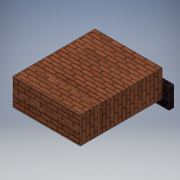
# Autodesk Inventor part: Камин
Saved by Autodesk Inventor 2019 (Build 230136000, 136)
## iProperties
Created: 2018-09-19
Part Number: Камин
Material: Кирпич, обычный, коричневый
Document SubType Name: Modeling
Designer: Андреев Н.Л.
Density: 1.95 g/cm^3
Appearance: Равномерная кладка — непрерывный ряд — оранжевый
Author: Андреев Н.Л.
Autodesk Inventor part; units mm, degrees
ref_plane "YZ Plane" through (0, 0, 0) normal (1, 0, 0) x (0, 1, 0)
ref_plane "XZ Plane" through (0, 0, 0) normal (0, 1, 0) x (-1, 0, 0)
ref_plane "XY Plane" through (0, 0, 0) normal (0, 0, 1) x (1, 0, 0)
sketch "Эскиз1" plane through (0, 0, 0) normal (0, 0, 1) x (1, 0, 0)
  line L0 (-750, -187.5) -> (750, -187.5)
  line L1 (750, -187.5) -> (750, 187.5)
  line L2 (750, 187.5) -> (-750, 187.5)
  line L3 (-750, 187.5) -> (-750, -187.5)
  line L4 (-750, -187.5) -> (750, 187.5) construction
  line L5 (750, -187.5) -> (-750, 187.5) construction
  point P0 (0, 0)
  dimension "d0" = 1500
  dimension "d1" = 375
  constraints: 12 end point, 2 midpoint, 2 parallel, 1 horizontal, 1 perpendicular
  measures "d0" distance of L2.end L1.end
  measures "d1" distance of L1.end L0.end
extrude "Выдавливание1" add sketch "Эскиз1" along normal blind 90
sketch "Эскиз2" plane through (0, 0, 90) normal (0, 0, 1) x (1, 0, 0)
  line L0 (-750, -187.5) -> (750, -187.5) construction
  line L1 (750, -187.5) -> (750, 187.5) construction
  line L2 (750, 187.5) -> (-750, 187.5) construction
  line L3 (-750, 187.5) -> (-750, -187.5) construction
  line L4 (-625, -62.5) -> (625, -62.5)
  line L5 (625, -62.5) -> (625, 437.5)
  line L6 (625, 437.5) -> (-625, 437.5)
  line L7 (-625, 437.5) -> (-625, -62.5)
  point P0 (0, 0)
  dimension "d4" = 1250
  dimension "d5" = 500
  dimension "d6" = 125
  dimension "d7" = 125
  dimension "d8" = 125
  constraints: 8 end point, 2 parallel, 1 horizontal, 1 perpendicular
  measures "d4" distance of L6.end L5.end
  measures "d5" distance of L5.end L4.end
  measures "d6" distance between parallel lines of L3 L7
  measures "d7" distance between parallel lines of L1 L5
  measures "d8" distance between parallel lines of L4 L0
extrude "Выдавливание2" add sketch "Эскиз2" along normal blind 1520 separate body
sketch "Эскиз3" plane through (-625, -62.5, 90) normal (0, -1, 0) x (1, 0, 0)
  line L0 (0, 0) -> (1250, 0) construction
  line L1 (1250, 0) -> (1250, 1520) construction
  line L2 (0, 1520) -> (1250, 1520) construction
  line L3 (0, 0) -> (0, 1520) construction
  line L4 (250, 80) -> (1000, 80)
  line L5 (1000, 80) -> (1000, 800)
  line L6 (1000, 800) -> (250, 800)
  line L7 (250, 800) -> (250, 80)
  point P0 (625, -90)
  dimension "d11" = 720
  dimension "d12" = 250
  dimension "d13" = 250
  dimension "d14" = 80
  constraints: 8 end point, 2 parallel, 1 horizontal, 1 perpendicular
  measures "d11" distance of L5.end L4.end
  measures "d12" distance between parallel lines of L1 L5
  measures "d13" distance between parallel lines of L3 L7
  measures "d14" distance between parallel lines of L0 L4
extrude "Выдавливание3" cut sketch "Эскиз3" against normal blind 375 bodies 2
sketch "Эскиз4" plane through (-625, -62.5, 90) normal (0, -1, 0) x (1, 0, 0)
  line L0 (1000, 800) -> (1000, 80) construction
  line L1 (1000, 80) -> (250, 80) construction
  line L2 (250, 80) -> (250, 800) construction
  line L3 (250, 800) -> (1000, 800) construction
  line L4 (0, 0) -> (1250, 0) construction
  line L5 (1250, 0) -> (1250, 1520) construction
  line L6 (0, 1520) -> (1250, 1520) construction
  line L7 (0, 0) -> (0, 1520) construction
  line L8 (223.236, 800) -> (1026.764, 800)
  line L9 (1026.764, 800) -> (1026.764, 1040) construction
  line L10 (1026.764, 1040) -> (223.236, 1040) construction
  line L11 (223.236, 1040) -> (223.236, 800) construction
  arc A0 (1092.9044, 906.0681) -> (157.0956, 906.0681) centre (625, 155.6985) ccw
  line L12 (223.236, 800) -> (157.0956, 906.0681)
  line L13 (1092.9044, 906.0681) -> (1026.764, 800)
  arc A1 (1026.764, 800) -> (223.236, 800) centre (625, 155.6985) ccw
  point P0 (625, -90)
  point P1 (625, 1040)
  dimension "d17" = 240
  dimension "d18" = 26.764
  dimension "d19" = 26.764
  dimension "d20" = 125
  constraints: 12 end point, 5 point on circle, 2 centre point, 2 parallel, 1 collinear, 1 concentric, 1 horizontal, 1 horizontal alignment, 1 line through centre, 1 midpoint, 1 perpendicular
  measures "d17" distance of L9.end L8.end
  measures "d18" distance between parallel lines of L2 L11
  measures "d19" distance between parallel lines of L0 L9
  measures "d20" distance of L8.start L12.end
extrude "Выдавливание4" cut sketch "Эскиз4" against normal blind 375 contours A1 L8 bodies 2
extrude "Выдавливание5" add sketch "Эскиз4" along normal blind 0.5 contours L12 A0 L13 A1 bodies 2
equation "\"d6\" = d7"
equation "\"d8\" = d7"
equation "\"d13\" = d12"
equation "\"d19\" = d18"
